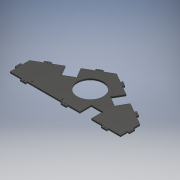
# Autodesk Inventor part: BA07
Saved by Autodesk Inventor 2017 (Build 210142000, 142)
## iProperties
Created: 2019-05-24
Part Number: BA07
Material: Polyethylene, High Density
Document SubType Name: Modeling
Designer: Dell
Density: 0.952 g/cm^3
Appearance: Smooth - Black
Mass: 784.258 g
Surface Area: 1599.12 cm^2
Volume: 823.801 cm^3
Author: Dell
Autodesk Inventor part; units mm, degrees
ref_plane "YZ Plane" through (0, 0, 0) normal (1, 0, 0) x (0, 1, 0)
ref_plane "XZ Plane" through (0, 0, 0) normal (0, 1, 0) x (-1, 0, 0)
ref_plane "XY Plane" through (0, 0, 0) normal (0, 0, 1) x (1, 0, 0)
sketch "Sketch1" plane through (0, 0, 0) normal (0, 0, 1) x (1, 0, 0)
  line L0 (0, 0) -> (0, 101.6)
  line L1 (0, 0) -> (525.78, 0)
  line L2 (525.78, 0) -> (525.78, 101.6)
  line L3 (525.78, 101.6) -> (262.89, 253.3796)
  line L4 (262.89, 253.3796) -> (0, 101.6)
  line L5 (7.62, 97.2006) -> (7.62, 7.62)
  line L6 (7.62, 7.62) -> (518.16, 7.62)
  line L7 (518.16, 7.62) -> (518.16, 97.2006)
  line L8 (518.16, 97.2006) -> (262.89, 244.5808)
  line L9 (262.89, 244.5808) -> (7.62, 97.2006)
  point P0 (262.89, 0)
  dimension "d0" = 101.6
  dimension "d1" = 525.78
  dimension "d2" = 120
  dimension "d3" = 7.62
  constraints: 20 end point, 2 perpendicular, 1 horizontal, 1 horizontal alignment, 1 midpoint, 1 vertical, 1 vertical alignment, 4 other
  measures "d0" distance of L0.start L0.end
  measures "d1" distance of L0.start L1.end
  measures "d2" angle of L0 L4
  measures "d3" distance between parallel lines of L4 L9
extrude "Extrusion1" add sketch "Sketch1" along normal blind 6.35 contours L9 L8 L7 L6 L5
sketch "Sketch2" plane through (0, 0, 6.35) normal (0, 0, 1) x (1, 0, 0)
  line L0 (7.62, 97.2006) -> (7.62, 7.62) projected
  line L1 (7.62, 64.8419) -> (1.27, 64.8419)
  line L2 (1.27, 64.8419) -> (1.27, 39.4419)
  line L3 (1.27, 39.4419) -> (7.62, 39.4419)
  line L4 (7.62, 39.4419) -> (7.62, 64.8419)
  line L5 (518.16, 64.8419) -> (524.51, 64.8419)
  line L6 (524.51, 64.8419) -> (524.51, 39.4419)
  line L7 (524.51, 39.4419) -> (518.16, 39.4419)
  line L8 (518.16, 39.4419) -> (518.16, 64.8419)
  line L9 (518.16, 7.62) -> (518.16, 97.2006) projected
  line L10 (7.62, 7.62) -> (518.16, 7.62) projected
  line L11 (62.69, 7.62) -> (88.09, 7.62)
  line L12 (88.09, 7.62) -> (88.09, 1.27)
  line L13 (88.09, 1.27) -> (62.69, 1.27)
  line L14 (62.69, 1.27) -> (62.69, 7.62)
  line L15 (250.19, 7.62) -> (275.59, 7.62)
  line L16 (275.59, 7.62) -> (275.59, 1.27)
  line L17 (275.59, 1.27) -> (250.19, 1.27)
  line L18 (250.19, 1.27) -> (250.19, 7.62)
  line L19 (437.69, 7.62) -> (463.09, 7.62)
  line L20 (463.09, 7.62) -> (463.09, 1.27)
  line L21 (463.09, 1.27) -> (437.69, 1.27)
  line L22 (437.69, 1.27) -> (437.69, 7.62)
  line L23 (75.39, 1.27) -> (450.39, 1.27) construction
  line L24 (48.4793, 120.7907) -> (45.3043, 126.29)
  line L25 (45.3043, 126.29) -> (67.3013, 138.99)
  line L26 (67.3013, 138.99) -> (70.4763, 133.4907)
  line L27 (70.4763, 133.4907) -> (48.4793, 120.7907)
  line L28 (200.0337, 208.2907) -> (196.8587, 213.79)
  line L29 (196.8587, 213.79) -> (218.8557, 226.49)
  line L30 (218.8557, 226.49) -> (222.0307, 220.9907)
  line L31 (222.0307, 220.9907) -> (200.0337, 208.2907)
  line L32 (262.89, 244.5808) -> (7.62, 97.2006) projected
  line L33 (56.3028, 132.64) -> (207.8572, 220.14) construction
  line L34 (132.08, 176.39) -> (135.255, 170.8907)
  line L35 (518.16, 97.2006) -> (262.89, 244.5808) projected
  line L36 (262.89, 244.5808) -> (262.89, 274.3369)
  line L37 (477.3007, 120.7907) -> (480.4757, 126.29)
  line L38 (480.4757, 126.29) -> (458.4787, 138.99)
  line L39 (458.4787, 138.99) -> (455.3037, 133.4907)
  line L40 (455.3037, 133.4907) -> (477.3007, 120.7907)
  line L41 (325.7463, 208.2907) -> (328.9213, 213.79)
  line L42 (328.9213, 213.79) -> (306.9243, 226.49)
  line L43 (306.9243, 226.49) -> (303.7493, 220.9907)
  line L44 (303.7493, 220.9907) -> (325.7463, 208.2907)
  line L45 (469.4772, 132.64) -> (317.9228, 220.14) construction
  line L46 (393.7, 176.39) -> (390.525, 170.8907)
  circle A0 centre (521.335, 52.1419) radius 2.25
  circle A1 centre (467.8897, 129.8903) radius 2.25
  circle A2 centre (450.39, 4.445) radius 2.25
  circle A3 centre (262.89, 4.445) radius 2.25
  circle A4 centre (75.39, 4.445) radius 2.25
  circle A5 centre (4.445, 52.1419) radius 2.25
  circle A6 centre (57.8903, 129.8903) radius 2.25
  circle A7 centre (209.4447, 217.3903) radius 2.25
  circle A8 centre (316.3353, 217.3903) radius 2.25
  line L47 (57.8903, 129.8903) -> (56.3028, 132.64) construction
  line L48 (57.8903, 129.8903) -> (68.8888, 136.2403) construction
  line L49 (198.4462, 211.0403) -> (209.4447, 217.3903) construction
  line L50 (209.4447, 217.3903) -> (207.8572, 220.14) construction
  line L51 (327.3338, 211.0403) -> (316.3353, 217.3903) construction
  line L52 (316.3353, 217.3903) -> (317.9228, 220.14) construction
  line L53 (456.8912, 136.2403) -> (467.8897, 129.8903) construction
  line L54 (467.8897, 129.8903) -> (469.4772, 132.64) construction
  line L55 (6.35, 97.9338) -> (6.35, 6.35) construction
  line L56 (6.35, 6.35) -> (519.43, 6.35) construction
  line L57 (519.43, 6.35) -> (519.43, 97.9338) construction
  line L58 (519.43, 97.9338) -> (262.89, 246.0473) construction
  line L59 (262.89, 246.0473) -> (6.35, 97.9338) construction
  point P0 (0, 0)
  point P1 (262.89, 7.62)
  point P2 (262.89, 1.27)
  point P3 (262.89, 7.62)
  point P4 (88.09, 4.445)
  point P5 (250.19, 4.445)
  point P6 (437.69, 4.445)
  point P7 (7.62, 52.4103)
  point P8 (4.445, 64.8419)
  point P9 (75.39, 7.62)
  point P10 (262.89, 7.62)
  point P11 (450.39, 7.62)
  point P12 (521.335, 64.8419)
  point P13 (6.35, 52.1419)
  point P14 (1.27, 52.1419)
  point P15 (519.43, 52.1419)
  point P16 (524.51, 52.1419)
  dimension "d6" = 6.35
  dimension "d7" = 25.4
  dimension "d8" = 6.35
  dimension "d9" = 25.4
  dimension "d10" = 25.4
  dimension "d11" = 6.35
  dimension "d12" = 25.4
  dimension "d13" = 6.35
  dimension "d14" = 25.4
  dimension "d15" = 6.35
  dimension "d16" = 375
  dimension "d17" = 25.4
  dimension "d18" = 6.35
  dimension "d19" = 6.35
  dimension "d20" = 25.4
  dimension "d21" = 175
  dimension "d28" = 4.5
  dimension "d29" = 4.5
  dimension "d30" = 4.5
  dimension "d31" = 4.5
  dimension "d32" = 4.5
  dimension "d33" = 4.5
  dimension "d34" = 4.5
  dimension "d35" = 4.5
  dimension "d36" = 4.5
  dimension "d99" = 1.27
  constraints: 110 end point, 24 midpoint, 16 perpendicular, 14 parallel, 12 symmetric about line, 9 centre point, 7 horizontal alignment, 7 point on line, 6 vertical alignment, 5 horizontal, 1 vertical, 12 other
  measures "d6" distance of L3.end L2.end
  measures "d7" distance of L2.end L1.end
  measures "d8" distance of L6.end L7.end
  measures "d9" distance of L5.end L6.end
  measures "d10" distance of L12.end L13.end
  measures "d11" distance of L11.end L12.end
  measures "d12" distance of L16.end L17.end
  measures "d13" distance of L15.end L16.end
  measures "d14" distance of L20.end L21.end
  measures "d15" distance of L19.end L20.end
  measures "d16" distance of L23.start L23.end
  measures "d17" distance of L28.end L29.end
  measures "d18" distance of L29.end L30.end
  measures "d19" distance of L24.start L24.end
  measures "d20" distance of L24.end L25.end
  measures "d21" distance of L33.start L33.end
  measures "d28" diameter of A0
  measures "d29" diameter of A1
  measures "d30" diameter of A2
  measures "d31" diameter of A3
  measures "d32" diameter of A4
  measures "d33" diameter of A5
  measures "d34" diameter of A6
  measures "d35" diameter of A7
  measures "d36" diameter of A8
  measures "d99" distance between parallel lines of L32 L59
extrude "Extrusion2" add sketch "Sketch2" against normal blind 6.35
sketch "Sketch3" plane through (0, 0, 6.35) normal (0, 0, 1) x (1, 0, 0)
  circle A0 centre (262.89, 122.6496) radius 60
  line L0 (250.19, 1.27) -> (275.59, 1.27) projected
  point P0 (0, 0)
  point P1 (262.89, 1.27)
  dimension "d24" = 120
  dimension "d25" = 121.3796
  constraints: 1 centre point, 1 midpoint, 1 vertical alignment
  measures "d24" diameter of A0
  measures "d25" distance from line of L0 A0.centre
extrude "Extrusion3" cut sketch "Sketch3" against normal through all
sketch "Sketch5" plane through (0, 0, 6.35) normal (0, 0, 1) x (1, 0, 0)
  line L0 (275.59, 7.62) -> (437.69, 7.62) projected
  line L1 (329.97, 7.62) -> (383.31, 7.62)
  line L2 (383.31, 7.62) -> (383.31, 60.96)
  line L3 (383.31, 60.96) -> (329.97, 60.96)
  line L4 (329.97, 60.96) -> (329.97, 7.62)
  point P0 (0, 0)
  point P1 (356.64, 7.62)
  dimension "d37" = 53.34
  dimension "d38" = 53.34
  constraints: 8 end point, 2 midpoint, 2 parallel, 1 horizontal, 1 perpendicular, 1 point on line
  measures "d37" distance of L3.end L2.end
  measures "d38" distance of L2.end L1.end
extrude "Extrusion4" cut sketch "Sketch5" against normal through all
sketch "Sketch6" plane through (0, 0, 6.35) normal (0, 0, 1) x (1, 0, 0)
  line L0 (158.3519, 184.2257) -> (185.0219, 138.0319)
  line L1 (185.0219, 138.0319) -> (138.8281, 111.3619)
  line L2 (138.8281, 111.3619) -> (112.1581, 157.5557)
  line L3 (112.1581, 157.5557) -> (158.3519, 184.2257)
  line L4 (455.3037, 133.4907) -> (325.7463, 208.2907) projected
  line L5 (413.6219, 157.5557) -> (386.9519, 111.3619)
  line L6 (386.9519, 111.3619) -> (340.7581, 138.0319)
  line L7 (340.7581, 138.0319) -> (367.4281, 184.2257)
  line L8 (367.4281, 184.2257) -> (413.6219, 157.5557)
  line L9 (200.0337, 208.2907) -> (70.4763, 133.4907) projected
  point P0 (0, 0)
  point P1 (135.255, 170.8907)
  point P2 (390.525, 170.8907)
  dimension "d41" = 53.34
  dimension "d42" = 53.34
  dimension "d43" = 53.34
  dimension "d44" = 53.34
  constraints: 16 end point, 4 midpoint, 4 parallel, 4 point on line, 2 perpendicular
  measures "d41" distance of L5.end L6.end
  measures "d42" distance of L5.start L5.end
  measures "d43" distance of L0.end L1.end
  measures "d44" distance of L0.start L0.end
extrude "Extrusion5" cut sketch "Sketch6" against normal through all
sketch "Sketch7" plane through (0, 0, 6.35) normal (0, 0, 1) x (1, 0, 0)
  line L0 (88.09, 7.62) -> (110.19, 7.62) construction
  line L1 (110.19, 7.62) -> (110.19, 27.62) construction
  line L2 (110.19, 27.62) -> (88.09, 27.62) construction
  line L3 (88.09, 27.62) -> (88.09, 7.62) construction
  line L4 (250.19, 7.62) -> (228.09, 7.62) construction
  line L5 (228.09, 7.62) -> (228.09, 27.62) construction
  line L6 (228.09, 27.62) -> (250.19, 27.62) construction
  line L7 (250.19, 27.62) -> (250.19, 7.62) construction
  circle A0 centre (99.14, 17.62) radius 3
  circle A1 centre (239.14, 17.62) radius 3
  point P0 (0, 0)
  point P1 (250.19, 7.62)
  point P2 (99.14, 27.62)
  point P3 (239.14, 27.62)
  point P4 (88.09, 17.62)
  point P5 (250.19, 17.62)
  dimension "d48" = 20
  dimension "d50" = 20
  dimension "d51" = 6
  dimension "d52" = 6
  dimension "d55" = 11.05
  dimension "d56" = 11.05
  constraints: 16 end point, 4 midpoint, 4 parallel, 3 coincident, 2 centre point, 2 horizontal, 2 horizontal alignment, 2 perpendicular, 2 vertical alignment, 1 point on line
  measures "d48" distance of L1.end L0.end
  measures "d50" distance of L4.end L5.end
  measures "d51" diameter of A0
  measures "d52" diameter of A1
  measures "d55" horizontal distance of point (88.09, 7.62) A0.centre
  measures "d56" horizontal distance of A1.centre point (250.19, 7.62)
extrude "Extrusion6" cut sketch "Sketch7" against normal through all
sketch "Sketch8" plane through (0, 0, 6.35) normal (0, 0, 1) x (1, 0, 0)
  circle A0 centre (5.3749, 67.087) radius 3.175
  circle A1 centre (5.3749, 37.1968) radius 3.175
  circle A2 centre (60.4449, 5.3749) radius 3.175
  circle A3 centre (90.3351, 5.3749) radius 3.175
  circle A4 centre (247.9449, 5.3749) radius 3.175
  circle A5 centre (277.8351, 5.3749) radius 3.175
  circle A6 centre (435.4449, 5.3749) radius 3.175
  circle A7 centre (465.3351, 5.3749) radius 3.175
  circle A8 centre (520.4051, 37.1968) radius 3.175
  circle A9 centre (520.4051, 67.087) radius 3.175
  circle A10 centre (480.3676, 121.6124) radius 3.175
  circle A11 centre (454.4819, 136.5575) radius 3.175
  circle A12 centre (328.8131, 209.1124) radius 3.175
  circle A13 centre (302.9275, 224.0575) radius 3.175
  circle A14 centre (222.8525, 224.0575) radius 3.175
  circle A15 centre (196.9669, 209.1124) radius 3.175
  circle A16 centre (71.2981, 136.5575) radius 3.175
  circle A17 centre (45.4124, 121.6124) radius 3.175
  line L0 (60.4449, 5.3749) -> (62.69, 7.62)
  line L1 (7.62, 7.62) -> (62.69, 7.62) projected
  line L2 (7.62, 97.2006) -> (7.62, 64.8419) projected
  line L3 (518.16, 64.8419) -> (520.4051, 67.087)
  line L4 (518.16, 64.8419) -> (524.51, 64.8419) projected
  line L5 (477.3007, 120.7907) -> (480.3676, 121.6124)
  line L6 (480.3676, 121.6124) -> (302.9275, 224.0575)
  line L7 (518.16, 97.2006) -> (477.3007, 120.7907) projected
  line L8 (367.4281, 184.2257) -> (325.7463, 208.2907) projected
  line L9 (45.3043, 126.29) -> (48.4793, 120.7907) projected
  line L10 (48.4793, 120.7907) -> (45.4124, 121.6124)
  line L11 (45.4124, 121.6124) -> (222.8525, 224.0575)
  line L12 (200.0337, 208.2907) -> (158.3519, 184.2257) projected
  line L13 (1.27, 64.8419) -> (7.62, 64.8419) projected
  circle A18 centre (99.14, 17.62) radius 3 projected
  circle A19 centre (239.14, 17.62) radius 3 projected
  circle A20 centre (75.39, 4.445) radius 2.25 projected
  circle A21 centre (262.89, 4.445) radius 2.25 projected
  circle A22 centre (450.39, 4.445) radius 2.25 projected
  circle A23 centre (4.445, 52.1419) radius 2.25 projected
  circle A24 centre (521.335, 52.1419) radius 2.25 projected
  circle A25 centre (57.8903, 129.8903) radius 2.25 projected
  circle A26 centre (209.4447, 217.3903) radius 2.25 projected
  circle A27 centre (467.8897, 129.8903) radius 2.25 projected
  circle A28 centre (316.3353, 217.3903) radius 2.25 projected
  circle A29 centre (262.89, 122.6496) radius 60 projected
  line L14 (158.3519, 184.2257) -> (185.0219, 138.0319) projected
  line L15 (185.0219, 138.0319) -> (138.8281, 111.3619) projected
  line L16 (138.8281, 111.3619) -> (112.1581, 157.5557) projected
  line L17 (112.1581, 157.5557) -> (70.4763, 133.4907) projected
  line L18 (70.4763, 133.4907) -> (67.3013, 138.99) projected
  line L19 (67.3013, 138.99) -> (45.3043, 126.29) projected
  line L20 (45.3043, 126.29) -> (48.4793, 120.7907) projected
  line L21 (48.4793, 120.7907) -> (7.62, 97.2006) projected
  line L22 (7.62, 97.2006) -> (7.62, 64.8419) projected
  line L23 (7.62, 64.8419) -> (1.27, 64.8419) projected
  line L24 (1.27, 64.8419) -> (1.27, 39.4419) projected
  line L25 (1.27, 39.4419) -> (7.62, 39.4419) projected
  line L26 (7.62, 39.4419) -> (7.62, 7.62) projected
  line L27 (7.62, 7.62) -> (62.69, 7.62) projected
  line L28 (62.69, 7.62) -> (62.69, 1.27) projected
  line L29 (62.69, 1.27) -> (88.09, 1.27) projected
  line L30 (88.09, 1.27) -> (88.09, 7.62) projected
  line L31 (88.09, 7.62) -> (250.19, 7.62) projected
  line L32 (250.19, 7.62) -> (250.19, 1.27) projected
  line L33 (250.19, 1.27) -> (275.59, 1.27) projected
  line L34 (275.59, 1.27) -> (275.59, 7.62) projected
  line L35 (275.59, 7.62) -> (329.97, 7.62) projected
  line L36 (329.97, 7.62) -> (329.97, 60.96) projected
  line L37 (329.97, 60.96) -> (383.31, 60.96) projected
  line L38 (383.31, 60.96) -> (383.31, 7.62) projected
  line L39 (383.31, 7.62) -> (437.69, 7.62) projected
  line L40 (437.69, 7.62) -> (437.69, 1.27) projected
  line L41 (437.69, 1.27) -> (463.09, 1.27) projected
  line L42 (463.09, 1.27) -> (463.09, 7.62) projected
  line L43 (463.09, 7.62) -> (518.16, 7.62) projected
  line L44 (518.16, 7.62) -> (518.16, 39.4419) projected
  line L45 (518.16, 39.4419) -> (524.51, 39.4419) projected
  line L46 (524.51, 39.4419) -> (524.51, 64.8419) projected
  line L47 (524.51, 64.8419) -> (518.16, 64.8419) projected
  line L48 (518.16, 64.8419) -> (518.16, 97.2006) projected
  line L49 (518.16, 97.2006) -> (477.3007, 120.7907) projected
  line L50 (480.4757, 126.29) -> (477.3007, 120.7907) projected
  line L51 (458.4787, 138.99) -> (480.4757, 126.29) projected
  line L52 (455.3037, 133.4907) -> (458.4787, 138.99) projected
  line L53 (455.3037, 133.4907) -> (413.6219, 157.5557) projected
  line L54 (413.6219, 157.5557) -> (386.9519, 111.3619) projected
  line L55 (386.9519, 111.3619) -> (340.7581, 138.0319) projected
  line L56 (340.7581, 138.0319) -> (367.4281, 184.2257) projected
  line L57 (367.4281, 184.2257) -> (325.7463, 208.2907) projected
  line L58 (325.7463, 208.2907) -> (328.9213, 213.79) projected
  line L59 (328.9213, 213.79) -> (306.9243, 226.49) projected
  line L60 (306.9243, 226.49) -> (303.7493, 220.9907) projected
  line L61 (303.7493, 220.9907) -> (262.89, 244.5808) projected
  line L62 (262.89, 244.5808) -> (222.0307, 220.9907) projected
  line L63 (222.0307, 220.9907) -> (218.8557, 226.49) projected
  line L64 (218.8557, 226.49) -> (196.8587, 213.79) projected
  line L65 (196.8587, 213.79) -> (200.0337, 208.2907) projected
  line L66 (200.0337, 208.2907) -> (158.3519, 184.2257) projected
  line L67 (247.9449, 5.3749) -> (90.3351, 5.3749)
  line L68 (90.3351, 5.3749) -> (90.3351, -0.9751)
  line L69 (90.3351, -0.9751) -> (60.4449, -0.9751)
  line L70 (60.4449, -0.9751) -> (60.4449, 5.3749)
  line L71 (60.4449, 5.3749) -> (5.3749, 5.3749)
  line L72 (5.3749, 5.3749) -> (5.3749, 37.1968)
  line L73 (5.3749, 37.1968) -> (-0.9751, 37.1968)
  line L74 (-0.9751, 37.1968) -> (-0.9751, 67.087)
  line L75 (-0.9751, 67.087) -> (5.3749, 67.087)
  line L76 (5.3749, 67.087) -> (5.3749, 98.4968)
  line L77 (5.3749, 98.4968) -> (45.4124, 121.6124)
  line L78 (45.4124, 121.6124) -> (42.2374, 127.1117)
  line L79 (42.2374, 127.1117) -> (68.1231, 142.0568)
  line L80 (68.1231, 142.0568) -> (71.2981, 136.5575)
  line L81 (71.2981, 136.5575) -> (112.9799, 160.6225)
  line L82 (112.9799, 160.6225) -> (139.6499, 114.4287)
  line L83 (139.6499, 114.4287) -> (181.9551, 138.8536)
  line L84 (181.9551, 138.8536) -> (155.2851, 185.0474)
  line L85 (155.2851, 185.0474) -> (196.9669, 209.1124)
  line L86 (196.9669, 209.1124) -> (193.7919, 214.6117)
  line L87 (193.7919, 214.6117) -> (219.6775, 229.5568)
  line L88 (219.6775, 229.5568) -> (222.8525, 224.0575)
  line L89 (222.8525, 224.0575) -> (262.89, 247.1732)
  line L90 (262.89, 247.1732) -> (302.9275, 224.0575)
  line L91 (302.9275, 224.0575) -> (306.1025, 229.5568)
  line L92 (306.1025, 229.5568) -> (331.9881, 214.6117)
  line L93 (331.9881, 214.6117) -> (328.8131, 209.1124)
  line L94 (328.8131, 209.1124) -> (370.4949, 185.0474)
  line L95 (370.4949, 185.0474) -> (343.8249, 138.8536)
  line L96 (343.8249, 138.8536) -> (386.1301, 114.4287)
  line L97 (386.1301, 114.4287) -> (412.8001, 160.6225)
  line L98 (412.8001, 160.6225) -> (454.4819, 136.5575)
  line L99 (454.4819, 136.5575) -> (457.6569, 142.0568)
  line L100 (457.6569, 142.0568) -> (483.5426, 127.1117)
  line L101 (483.5426, 127.1117) -> (480.3676, 121.6124)
  line L102 (480.3676, 121.6124) -> (520.4051, 98.4968)
  line L103 (520.4051, 98.4968) -> (520.4051, 67.087)
  line L104 (520.4051, 67.087) -> (526.7551, 67.087)
  line L105 (526.7551, 67.087) -> (526.7551, 37.1968)
  line L106 (526.7551, 37.1968) -> (520.4051, 37.1968)
  line L107 (520.4051, 37.1968) -> (520.4051, 5.3749)
  line L108 (520.4051, 5.3749) -> (465.3351, 5.3749)
  line L109 (465.3351, 5.3749) -> (465.3351, -0.9751)
  line L110 (465.3351, -0.9751) -> (435.4449, -0.9751)
  line L111 (435.4449, -0.9751) -> (435.4449, 5.3749)
  line L112 (435.4449, 5.3749) -> (381.0649, 5.3749)
  line L113 (381.0649, 5.3749) -> (381.0649, 58.7149)
  line L114 (381.0649, 58.7149) -> (332.2151, 58.7149)
  line L115 (332.2151, 58.7149) -> (332.2151, 5.3749)
  line L116 (332.2151, 5.3749) -> (277.8351, 5.3749)
  line L117 (277.8351, 5.3749) -> (277.8351, -0.9751)
  line L118 (277.8351, -0.9751) -> (247.9449, -0.9751)
  line L119 (247.9449, -0.9751) -> (247.9449, 5.3749)
  point P0 (0, 0)
  dimension "d57" = 6.35
  dimension "d58" = 6.35
  dimension "d59" = 6.35
  dimension "d60" = 6.35
  dimension "d61" = 6.35
  dimension "d62" = 6.35
  dimension "d63" = 6.35
  dimension "d64" = 6.35
  dimension "d65" = 6.35
  dimension "d66" = 6.35
  dimension "d67" = 6.35
  dimension "d68" = 6.35
  dimension "d69" = 6.35
  dimension "d70" = 6.35
  dimension "d71" = 6.35
  dimension "d72" = 6.35
  dimension "d73" = 6.35
  dimension "d74" = 6.35
  dimension "d75" = 45
  dimension "d77" = 45
  dimension "d78" = 45
  dimension "d79" = 45
  constraints: 118 end point, 5 horizontal alignment, 4 point on line, 2 parallel, 2 vertical alignment, 1 coincident, 1 perpendicular, 106 other
  measures "d75" angle of L1 L0
  measures "d77" angle of L4 L3
  measures "d78" angle of L5 L7
  measures "d79" angle of L9 L10
extrude "Extrusion7" cut sketch "Sketch8" along normal through all both and the other way through all contours L2 A0 | L13 A0 L75 L76 L2 | A0 L13 | A0 L76 L75 | L21 A17 | A17 L77 L10 L21 | L25 L26 A1 L72 L73 | A1 L25 | A17 L78 L77 | L9 L11 A17 | L10 L11 L9 | L73 L72 A1 | A1 L26 | A17 L9 L11 L78 | L9 A17 L11 | L71 L70 A2 | A2 L1 L0 L71 | A2 L1 | L80 L11 L18 A16 | A16 L11 L80 | L70 L0 L28 A2 | A2 L28 | L18 L11 A16 | A16 L17 L18 L11 | L11 L18 A16 | L17 A16 | L68 L67 A3 | A3 L30 L31 L67 L68 | L11 L65 L12 A15 | A15 L86 L11 | A3 L30 | A15 L65 L11 L86 | L12 A15 | A3 L31 | L67 L119 A4 | A4 L31 L32 L119 L67 | A15 L11 L65 | L65 L11 A15 | A4 L31 | A4 L32 | L88 L11 L63 A14 | A14 L89 L88 | L63 L11 A14 | A14 L62 L63 L11 L89 | L117 L116 A5 | A5 L34 L35 L116 L117 | L11 L63 A14 | A5 L34 | L62 A14 | L90 L6 L60 L61 A13 | A13 L91 L90 | A5 L35 | A13 L60 L6 L91 | L61 A13 | A13 L6 L60 | L60 L6 A13 | L93 L6 L58 A12 | A12 L6 L93 | L112 L111 A6 | A6 L39 L40 L111 L112 | L58 L6 A12 | L6 A12 L8 L58 | A6 L39 | L6 L58 A12 | A6 L40 | L8 A12 | L109 L108 A7 | A7 L42 L43 L108 L109 | L6 L52 L53 A11 | A11 L99 L6 | A7 L42 | A11 L52 L6 L99 | L53 A11 | A7 L43 | A11 L6 L52 | L52 L6 A11 | L107 L106 A8 | A8 L44 L45 L106 L107 | A8 L44 | L101 L6 L50 A10 | A10 L102 L101 | A8 L45 | L50 L6 A10 | L102 A10 L7 L5 | L5 L50 L6 | L6 L50 A10 | L7 A10 | L104 L103 A9 | A9 L4 L3 L104 | A9 L4 | L103 L3 L48 A9 | A9 L48
sketch "Sketch9" plane through (0, 0, 6.35) normal (0, 0, 1) x (1, 0, 0)
  circle A0 centre (139.6499, 114.4287) radius 3.175
  circle A1 centre (181.9551, 138.8536) radius 3.175
  circle A2 centre (343.8249, 138.8536) radius 3.175
  circle A3 centre (386.1301, 114.4287) radius 3.175
  circle A4 centre (332.2151, 58.7149) radius 3.175
  circle A5 centre (381.0649, 58.7149) radius 3.175
  line L0 (138.8281, 111.3619) -> (112.1581, 157.5557) projected
  line L1 (138.8281, 111.3619) -> (139.6499, 114.4287)
  line L2 (139.6499, 114.4287) -> (181.9551, 138.8536)
  line L3 (340.7581, 138.0319) -> (386.9519, 111.3619) projected
  line L4 (340.7581, 138.0319) -> (343.8249, 138.8536)
  line L5 (343.8249, 138.8536) -> (386.1301, 114.4287)
  line L6 (383.31, 60.96) -> (329.97, 60.96) projected
  line L7 (329.97, 60.96) -> (332.2151, 58.7149)
  line L8 (332.2151, 58.7149) -> (381.0649, 58.7149)
  line L9 (185.0219, 138.0319) -> (138.8281, 111.3619) projected
  point P0 (0, 0)
  dimension "d82" = 6.35
  dimension "d86" = 6.35
  dimension "d87" = 6.35
  dimension "d88" = 6.35
  dimension "d89" = 6.35
  dimension "d90" = 6.35
  dimension "d83" = 45
  dimension "d84" = 45
  dimension "d85" = 45
  constraints: 12 end point, 2 parallel, 1 horizontal, 18 other
  measures "d83" angle of L9 L1
  measures "d84" angle of L3 L4
  measures "d85" angle of L6 L7
extrude "Extrusion8" cut sketch "Sketch9" against normal through all contours A0 L9 L1 L2 | L2 L1 L0 A0 | A0 L9 | L0 A0 | A1 L9 | L9 A1 | A2 L5 L4 | L3 A2 | L4 L5 A2 L3 | A3 L3 | L3 A3 | L7 L8 A4 | A4 L6 | L6 A4 L8 L7 | A5 L6 | A5 L6
sketch "Sketch11" plane through (0, 0, 6.35) normal (0, 0, 1) x (1, 0, 0)
  line L0 (1.27, 39.4419) -> (-1.27, 39.4419)
  line L1 (-1.27, 39.4419) -> (-1.27, 64.8419)
  line L2 (-1.27, 64.8419) -> (1.27, 64.8419)
  line L3 (1.27, 64.8419) -> (1.27, 39.4419)
  line L4 (88.09, 1.27) -> (62.69, 1.27) projected
  line L5 (62.69, 1.27) -> (88.09, 1.27)
  line L6 (88.09, 1.27) -> (88.09, -1.27)
  line L7 (88.09, -1.27) -> (62.69, -1.27)
  line L8 (62.69, -1.27) -> (62.69, 1.27)
  line L9 (250.19, 3.1299) -> (250.19, 1.27) projected
  line L10 (250.19, 1.27) -> (275.59, 1.27)
  line L11 (275.59, 1.27) -> (275.59, -1.27)
  line L12 (275.59, -1.27) -> (250.19, -1.27)
  line L13 (250.19, -1.27) -> (250.19, 1.27)
  line L14 (46.2342, 124.6793) -> (45.3043, 126.29) projected
  line L15 (45.3043, 126.29) -> (44.0343, 128.4897)
  line L16 (44.0343, 128.4897) -> (66.0313, 141.1897)
  line L17 (66.0313, 141.1897) -> (67.3013, 138.99)
  line L18 (67.3013, 138.99) -> (45.3043, 126.29)
  line L19 (219.7857, 224.8793) -> (218.8557, 226.49) projected
  line L20 (218.8557, 226.49) -> (217.5857, 228.6897)
  line L21 (217.5857, 228.6897) -> (195.5887, 215.9897)
  line L22 (195.5887, 215.9897) -> (196.8587, 213.79)
  line L23 (196.8587, 213.79) -> (218.8557, 226.49)
  line L24 (299.8607, 223.2358) -> (262.89, 244.5808) projected
  line L25 (262.89, 244.5808) -> (262.89, 266.7054)
  line L26 (524.51, 39.4419) -> (527.05, 39.4419)
  line L27 (527.05, 39.4419) -> (527.05, 64.8419)
  line L28 (527.05, 64.8419) -> (524.51, 64.8419)
  line L29 (524.51, 64.8419) -> (524.51, 39.4419)
  line L30 (437.69, 1.27) -> (463.09, 1.27)
  line L31 (463.09, 1.27) -> (437.69, 1.27)
  line L32 (437.69, 1.27) -> (437.69, -1.27)
  line L33 (437.69, -1.27) -> (463.09, -1.27)
  line L34 (463.09, -1.27) -> (463.09, 1.27)
  line L35 (479.5458, 124.6793) -> (480.4757, 126.29)
  line L36 (480.4757, 126.29) -> (481.7457, 128.4897)
  line L37 (481.7457, 128.4897) -> (459.7487, 141.1897)
  line L38 (459.7487, 141.1897) -> (458.4787, 138.99)
  line L39 (458.4787, 138.99) -> (480.4757, 126.29)
  line L40 (305.9943, 224.8793) -> (306.9243, 226.49)
  line L41 (306.9243, 226.49) -> (308.1943, 228.6897)
  line L42 (308.1943, 228.6897) -> (330.1913, 215.9897)
  line L43 (330.1913, 215.9897) -> (328.9213, 213.79)
  line L44 (328.9213, 213.79) -> (306.9243, 226.49)
  point P0 (0, 0)
  point P1 (525.78, 0)
  dimension "d93" = 2.54
  dimension "d94" = 2.54
  dimension "d95" = 2.54
  dimension "d96" = 2.54
  constraints: 80 end point, 22 symmetric about line, 10 parallel, 7 coincident, 6 perpendicular, 3 horizontal, 1 collinear, 1 point on line, 1 vertical
  measures "d93" distance of L19.end L20.end
  measures "d94" distance of L16.end L17.end
  measures "d95" distance of L1.end L2.end
  measures "d96" distance of L7.end L4.end
extrude "Extrusion9" add sketch "Sketch11" against normal blind 6.35
equation "\"d3\" = Panel_Thickness + Fit_Tolerance"
equation "\"d4\" = Panel_Thickness"
equation "\"d6\" = d11"
equation "\"d8\" = d11"
equation "\"d9\" = d7"
equation "\"d10\" = d7"
equation "\"d11\" = Panel_Thickness"
equation "\"d12\" = d7"
equation "\"d13\" = d11"
equation "\"d14\" = d7"
equation "\"d15\" = d13"
equation "\"d17\" = d7"
equation "\"d18\" = d11"
equation "\"d19\" = d11"
equation "\"d20\" = d7"
equation "\"d99\" = Fit_Tolerance"
equation "\"d22\" = Panel_Thickness"
equation "\"d41\" = d43"
equation "\"d42\" = d41"
equation "\"d44\" = d43"
equation "\"d57\" = Tool_Dia"
equation "\"d58\" = d57"
equation "\"d59\" = d58"
equation "\"d60\" = d59"
equation "\"d61\" = d60"
equation "\"d62\" = d61"
equation "\"d63\" = d62"
equation "\"d64\" = d57"
equation "\"d65\" = d63"
equation "\"d66\" = d63"
equation "\"d67\" = d65"
equation "\"d68\" = d65"
equation "\"d69\" = d68"
equation "\"d70\" = d69"
equation "\"d71\" = d70"
equation "\"d72\" = d71"
equation "\"d73\" = d72"
equation "\"d74\" = d73"
equation "\"d82\" = Tool_Dia"
equation "\"d86\" = d82"
equation "\"d87\" = d86"
equation "\"d88\" = d87"
equation "\"d89\" = d88"
equation "\"d90\" = d88"
equation "\"d93\" = 2 * Fit_Tolerance"
equation "\"d94\" = 2 * Fit_Tolerance"
equation "\"d95\" = 2 * Fit_Tolerance"
equation "\"d96\" = 2 * Fit_Tolerance"
equation "\"d97\" = Panel_Thickness"
equation "\"Panel_Thickness\" = 6.35"
equation "\"Fit_Tolerance\" = 1.27"
equation "\"Tool_Dia\" = 6.35"
body "Solid1"
